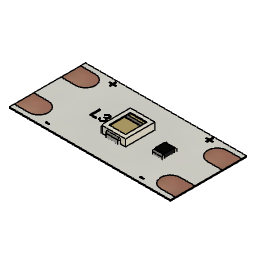
Shoulder LEDs v17 (Autodesk Fusion 360 archive; units mm, degrees)
design "LED D100"
Autodesk Fusion 360 part; units mm, degrees
sketch "Sketch1" plane through (0, 0, 0) normal (0, 0, 1) x (1, 0, 0)
  line L0 (0, 0) -> (16.5, 0)
  line L1 (16.5, 0) -> (16.5, 7.8)
  line L2 (0, 0) -> (0, 7.8)
  line L3 (16.5, 7.8) -> (0, 7.8)
  line L4 (8.25, 7.8) -> (8.25, 0) construction
  line L5 (0, 3.9) -> (16.5, 3.9) construction
  line L6 (8.25, 3.9) -> (8.25, 5.4) construction
  line L7 (8.25, 5.4) -> (8.25, 2.4) construction
  line L8 (8.25, 5.4) -> (7, 5.4) construction
  line L9 (7, 5.4) -> (9.5, 5.4)
  line L10 (9.5, 5.4) -> (9.5, 2.4)
  line L11 (9.5, 2.4) -> (7, 2.4)
  line L12 (7, 2.4) -> (7, 5.4)
  line L13 (7, 2.4) -> (9.5, 5.4) construction
  line L14 (7, 2.4) -> (7.064, 2.4768) construction
  line L15 (7.064, 2.4768) -> (7.1562, 2.4)
  line L16 (7.1562, 2.4) -> (7, 2.5302)
  line L17 (9.5, 3.9) -> (11.5, 3.9) construction
  line L18 (11.5, 3.9) -> (11.5, 4.65)
  line L19 (11.5, 4.65) -> (11.5, 3.15)
  line L20 (11.5, 3.15) -> (12.5, 3.15)
  line L21 (12.5, 3.15) -> (12.5, 4.65)
  line L22 (12.5, 4.65) -> (11.5, 4.65)
  line L23 (11.5, 3.15) -> (11.5, 3.4)
  line L24 (11.5, 4.65) -> (11.5, 4.4)
  line L25 (11.5, 4.4) -> (12.5, 4.4)
  line L26 (11.5, 3.4) -> (12.5, 3.4)
  line L27 (0, 7.8) -> (0, 7.3)
  line L28 (0, 7.3) -> (0, 5.3)
  line L29 (0, 0) -> (0, 0.5)
  line L30 (0, 0.5) -> (0, 2.5)
  line L31 (0, 7.3) -> (2.5, 7.3)
  line L32 (0, 0.5) -> (2.5, 0.5)
  line L33 (0, 2.5) -> (2.5, 2.5)
  line L34 (0, 5.3) -> (2.5, 5.3)
  line L35 (2.5, 0.5) -> (1.5, 0.5) construction
  line L36 (1.5, 0.5) -> (1.5, 7.3) construction
  line L37 (1.5, 5.3) -> (1.5, 7.3) construction
  circle A0 centre (1.5, 6.3) radius 1
  line L38 (1.5, 0.5) -> (1.5, 2.5) construction
  circle A1 centre (1.5, 1.5) radius 1
  line L39 (2.5, 0.5) -> (16.5, 0.5) construction
  line L40 (2.5, 5.3) -> (16.5, 5.3) construction
  line L41 (2.5, 7.3) -> (16.5, 7.3) construction
  line L42 (2.5, 2.5) -> (16.5, 2.5) construction
  line L43 (16.5, 0.5) -> (14, 0.5)
  line L44 (14, 0.5) -> (14, 7.8) construction
  line L45 (16.5, 7.3) -> (14, 7.3)
  line L46 (16.5, 5.3) -> (14, 5.3)
  line L47 (16.5, 2.5) -> (14, 2.5)
  line L48 (14, 2.5) -> (15, 2.5) construction
  line L49 (15, 2.5) -> (15, 0.5) construction
  line L50 (15, 2.5) -> (15, 7.3) construction
  line L51 (15, 7.3) -> (15, 5.3) construction
  circle A2 centre (15, 1.5) radius 1
  circle A3 centre (15, 6.3) radius 1
  line L52 (8.25, 2.4) -> (8.25, 2.25) construction
  line L53 (8.25, 2.25) -> (7.5, 2.25)
  line L54 (7.5, 2.25) -> (9, 2.25)
  line L55 (9, 2.25) -> (9, 5.4) construction
  line L56 (9, 5.4) -> (9, 5.55) construction
  line L57 (9, 5.55) -> (7.5, 5.55)
  line L58 (7.5, 2.25) -> (7.65, 2.25) construction
  line L59 (7.65, 2.25) -> (7.65, 2.4) construction
  circle A4 centre (7.65, 2.4) radius 0.15
  line L60 (9, 2.4) -> (8.85, 2.4) construction
  circle A5 centre (8.85, 2.4) radius 0.15
  line L61 (8.85, 2.4) -> (8.85, 5.4) construction
  line L62 (7.65, 2.4) -> (7.625, 5.4) construction
  circle A6 centre (7.625, 5.4) radius 0.15
  circle A7 centre (8.85, 5.4) radius 0.15
  dimension "d1" = 16.5
  dimension "d2" = 7.8
  dimension "d4" = 3
  dimension "d8" = 2.5
  dimension "d13" = 0.1
  dimension "d16" = 2
  dimension "d18" = 1.5
  dimension "d19" = 1
  dimension "d30" = 0.5
  dimension "d31" = 2
  dimension "d32" = 0.5
  dimension "d33" = 2
  dimension "d34" = 2.5
  dimension "d35" = 2.5
  dimension "d36" = 1
  dimension "d37" = 2
  dimension "d38" = 2.5
  dimension "d39" = 1
  dimension "d40" = 2
  dimension "d41" = 2
  dimension "d44" = 0.15
  dimension "d45" = 0.15
  dimension "d46" = 1.5
  dimension "d47" = 0.15
  dimension "d48" = 0.15
  dimension "d49" = 0.3
  dimension "d50" = 0.3
  dimension "d51" = 0.3
  constraint coincident L0.start L2.start
  constraint horizontal L0
  constraint perpendicular L0 L1
  constraint perpendicular L0 L2
  constraint perpendicular L2 L3
  constraint midpoint L3 L4.start
  constraint midpoint L0 L4.end
  constraint midpoint L2 L5.start
  constraint midpoint L1 L5.end
  constraint midpoint L5 L6.start
  constraint perpendicular L5 L6
  constraint perpendicular L5 L7
  constraint perpendicular L4 L8
  constraint parallel L8 L9
  constraint perpendicular L5 L10
  constraint perpendicular L10 L11
  constraint parallel L13 L14
  constraint coincident L11 L15.end
  constraint perpendicular L13 L15
  constraint coincident L12 L16.end
  constraint perpendicular L13 L16
  constraint midpoint L10 L17.start
  constraint perpendicular L10 L17
  constraint perpendicular L17 L18
  constraint perpendicular L5 L19
  constraint perpendicular L19 L20
  constraint perpendicular L20 L21
  constraint perpendicular L20 L23
  constraint perpendicular L22 L24
  constraint coincident L21 L25.end
  constraint perpendicular L21 L25
  constraint coincident L21 L26.end
  constraint perpendicular L21 L26
  constraint perpendicular L3 L27
  constraint parallel L2 L28
  constraint perpendicular L0 L29
  constraint parallel L2 L30
  constraint perpendicular L2 L31
  constraint perpendicular L30 L32
  constraint perpendicular L30 L33
  constraint perpendicular L2 L34
  constraint parallel L32 L35
  constraint coincident L31 L36.end
  constraint perpendicular L31 L36
  constraint coincident L36 L37.start
  constraint coincident L34 L37.start
  constraint midpoint L37 A0.centre
  constraint coincident L37.start A0
  constraint coincident L36 L38.end
  constraint midpoint L38 A1.centre
  constraint coincident L1 L39.end
  constraint perpendicular L1 L39
  constraint coincident L1 L40.end
  constraint perpendicular L1 L40
  constraint coincident L1 L41.end
  constraint perpendicular L1 L41
  constraint coincident L1 L42.end
  constraint perpendicular L1 L42
  constraint perpendicular L1 L43
  constraint coincident L3 L44.end
  constraint perpendicular L3 L44
  constraint coincident L44 L45.end
  constraint coincident L41 L45.end
  constraint coincident L44 L46.end
  constraint coincident L40 L46.end
  constraint coincident L44 L47.end
  constraint coincident L42 L47.end
  constraint perpendicular L44 L48
  constraint coincident L43 L49.end
  constraint coincident L45 L50.end
  constraint coincident L46 L51.end
  constraint coincident L50 L51.end
  constraint midpoint L49 A2.centre
  constraint midpoint L51 A3.centre
  constraint perpendicular L11 L52
  constraint perpendicular L52 L53
  constraint perpendicular L52 L54
  constraint coincident L9 L55.end
  constraint perpendicular L9 L55
  constraint perpendicular L9 L56
  constraint perpendicular L56 L57
  constraint parallel L54 L58
  constraint coincident L11 L59.end
  constraint perpendicular L11 L59
  constraint coincident L59.end A4.centre
  constraint coincident L58.end A4
  constraint coincident L55 L60.start
  constraint coincident L11 L60.start
  constraint perpendicular L55 L60
  constraint coincident L60.end A5.centre
  constraint perpendicular L40 L61
  constraint midpoint L8 L62.end
  constraint coincident L62.end A6.centre
  constraint coincident L61.end A7.centre
  measures "d1" distance of L0.start L0.end
  measures "d2" distance of L0.end L1.end
  measures "d4" distance of L6.end L7.end
  measures "d8" distance of L10.end L11.end
  measures "d13" distance of L11.end L14.end
  measures "d16" distance of L17.start L17.end
  measures "d18" distance of L18.end L19.end
  measures "d19" distance of L19.end L20.end
  measures "d30" distance of L2.end L27.end
  measures "d31" distance of L27.end L28.end
  measures "d32" distance of L0.start L29.end
  measures "d33" distance of L29.end L30.end
  measures "d34" distance of L27.end L31.end
  measures "d35" distance of L29.end L32.end
  measures "d36" distance of L32.end L35.end
  measures "d37" diameter of A1
  measures "d38" distance of L39.end L43.end
  measures "d39" distance of L47.end L48.end
  measures "d40" diameter of A2
  measures "d41" diameter of A3
  measures "d44" distance of L7.end L52.end
  measures "d45" distance of L55.end L56.end
  measures "d46" distance of L56.end L57.end
  measures "d47" distance of L53.end L58.end
  measures "d48" distance of L60.start L60.end
  measures "d49" diameter of A5
  measures "d50" diameter of A6
  measures "d51" diameter of A7
extrude "Extrude8" add sketch "Sketch1" along normal blind 0.6 contours L9 A7 | L9 L57 A6 A7 | L9 A6 | L11 A5 | L11 L53 L54 A4 A5 | L11 A4 picked at (8.7907, 5.4648) picked at (7.6552, 5.4726) picked at (8.8359, 2.352) picked at (7.6439, 2.325) makes body 1 at (8, 2.4, 0.4) makes body 2 at (7.9833, 5.4, 0.4)
extrude "Extrude5" add sketch "Sketch1" along normal blind 0.45 separate body contours L18 L19 L21 L22 L24 L25 | L19 L20 L21 L23 L26 makes body 3 at (11.8333, 3.4, 0.15) makes body 4 at (11.8333, 4.4, 0.15)
extrude "Extrude4" add sketch "Sketch1" along normal blind 0.5 separate body contours L18 L19 L21 L25 L26 makes body 5
extrude "Extrude3" add sketch "Sketch1" along normal blind 0.7 separate body contours L11 L12 L15 L16 makes body 6
extrude "Extrude2" add sketch "Sketch1" along normal blind 0.8 separate body contours L9 A7 | L9 L10 L11 L12 L15 L16 A4 A5 A6 A7 | L9 A6 | L11 A5 | L11 A4 picked at (8.8017, 5.3778) picked at (7.669, 5.3354) picked at (8.875, 2.4433) picked at (7.6077, 2.4878) makes body 7
extrude "Extrude1" add sketch "Sketch1" along normal blind 0.1 separate body contours L0 L1 L2 L3 L27 L29 L31 L32 L33 L34 A0 A1 L43 L45 L46 L47 A2 A3 | L9 A7 | L9 L57 A6 A7 | L9 A6 | L11 A5 | L11 L53 L54 A4 A5 | L11 A4 | L18 L19 L21 L25 L26 | L18 L19 L21 L22 L24 L25 | L19 L20 L21 L23 L26 picked at (8.7907, 5.4648) picked at (7.6552, 5.4726) picked at (8.8359, 2.352) picked at (7.6439, 2.325) makes body 8
sketch "Sketch2" plane through (0, 0, 0.8) normal (0, 0, 1) x (-1, 0, 0)
  line L0 (-7.1562, -2.4) -> (-9.5, -2.4)
  line L1 (-9.5, -2.4) -> (-9.5, -5.4)
  line L2 (-9.5, -5.4) -> (-7, -5.4)
  line L3 (-7, -5.4) -> (-7, -2.5302)
  line L4 (-7, -2.5302) -> (-7.1562, -2.4)
  line L5 (-9.1, -5) -> (-7.4, -5)
  line L6 (-7.4, -5) -> (-7.4, -2.8)
  line L7 (-7.4, -2.8) -> (-9.1, -2.8)
  line L8 (-9.1, -2.8) -> (-9.1, -5)
  line L9 (-9.1, -5) -> (-9.1, -4.7)
  line L10 (-9.1, -4.7) -> (-7.4, -4.7)
  line L11 (-7.4, -4.7) -> (-7.4, -4.4)
  line L12 (-7.4, -4.4) -> (-9.1, -4.4)
  dimension "d27" = -0.4
  dimension "d82" = 0.3
  dimension "d83" = 0.3
  constraint perpendicular L5 L9
  constraint coincident L6 L10.end
  constraint perpendicular L6 L10
  constraint perpendicular L10 L11
  constraint coincident L8 L12.end
  constraint perpendicular L8 L12
  measures "d82" distance of L5.start L9.end
  measures "d83" distance of L10.end L11.end
extrude "Extrude17" cut sketch "Sketch2" against normal blind 0.05 contours L6 L8 L10 L11 L12 bodies 7
extrude "Extrude16" cut sketch "Sketch2" against normal blind 0.1 contours L5 L6 L8 L9 L10 | L6 L7 L8 L12 bodies 7
extrude "Extrude7" add sketch "Sketch1" along normal blind 0.09 contours L2 L30 L32 L33 A1 | L1 L43 L47 A2 | A1 | A2 | L2 L28 L31 L34 A0 | L1 L45 L46 A3 | A0 | A3 bodies 8
fillet "Fillet1" radius 0.15 3 edges at (7.5439, 2.2939, 0.6) (8.25, 2.25, 0.6) (8.9561, 2.2939, 0.6) on bodies 1
fillet "Fillet2" radius 0.15 3 edges at (8.9561, 5.5061, 0.6) (8.2375, 5.55, 0.6) (7.5189, 5.5061, 0.6) on bodies 2
fillet "Fillet3" radius 0.15 2 edges at (12, 3.15, 0.45) (12, 4.65, 0.45) on bodies 3 4
sketch "Sketch3" plane through (0, 0, 0.1) normal (0, 0, 1) x (-1, 0, 0)
  line L0 (-9.5, -2.4) -> (-7, -2.4)
  line L1 (-7, -2.4) -> (-7, -5.4)
  line L2 (-7, -5.4) -> (-9.5, -5.4)
  line L3 (-9.5, -5.4) -> (-9.5, -2.4)
  line L4 (-16.5, -7.8) -> (0, -7.8)
  line L5 (0, -7.8) -> (0, -7.3)
  line L6 (0, -7.3) -> (-1.5, -7.3)
  arc A0 (-1.5, -5.3) -> (-1.5, -7.3) centre (-1.5, -6.3) ccw
  line L7 (-1.5, -5.3) -> (0, -5.3)
  line L8 (0, -5.3) -> (0, -2.5)
  line L9 (0, -2.5) -> (-1.4999, -2.5)
  arc A1 (-1.5, -0.5) -> (-1.4999, -2.5) centre (-1.5, -1.5) ccw
  line L10 (-1.5, -0.5) -> (0, -0.5)
  line L11 (0, -0.5) -> (0, 0)
  line L12 (0, 0) -> (-16.5, 0)
  line L13 (-16.5, 0) -> (-16.5, -0.5)
  line L14 (-16.5, -0.5) -> (-15.0001, -0.5)
  arc A2 (-15, -2.5) -> (-15.0001, -0.5) centre (-15, -1.5) ccw
  line L15 (-15, -2.5) -> (-16.5, -2.5)
  line L16 (-16.5, -2.5) -> (-16.5, -5.3)
  line L17 (-16.5, -5.3) -> (-15.0003, -5.3)
  arc A3 (-15, -7.3) -> (-15.0003, -5.3) centre (-15, -6.3) ccw
  line L18 (-15, -7.3) -> (-16.5, -7.3)
  line L19 (-16.5, -7.3) -> (-16.5, -7.8)
  line L20 (-2.9593, -6.3608) -> (-4.4543, -6.3608) construction
  line L21 (-4.4543, -6.3608) -> (-4.4543, -7.6424) construction
  line L22 (-4.4543, -7.6424) -> (-2.9593, -7.6424) construction
  line L23 (-2.9593, -7.6424) -> (-2.9593, -6.3608) construction
  dimension "d60" = 1
  text T0 "+\n" font "Arial" height 1 align left top in box 1.4949 x 1.2816 at (-2.9593, -6.3608) x (-1, 0) y (0, -1) spacing 1 kerned
extrude "Extrude9" add sketch "Sketch3" along normal blind 0.01 text T0 bodies 8
sketch "Sketch4" plane through (0, 0, 0.1) normal (0, 0, 1) x (-1, 0, 0)
  line L0 (-3.2315, -6.9814) -> (-3.2315, -7.2556)
  line L1 (-3.2315, -7.2556) -> (-2.9593, -7.2556)
  line L2 (-2.9593, -7.2556) -> (-2.9593, -7.3702)
  line L3 (-2.9593, -7.3702) -> (-3.2315, -7.3702)
  line L4 (-3.2315, -7.3702) -> (-3.2315, -7.6424)
  line L5 (-3.2315, -7.6424) -> (-3.3474, -7.6424)
  line L6 (-3.3474, -7.6424) -> (-3.3474, -7.3702)
  line L7 (-3.3474, -7.3702) -> (-3.6196, -7.3702)
  line L8 (-3.6196, -7.3702) -> (-3.6196, -7.2556)
  line L9 (-3.6196, -7.2556) -> (-3.3474, -7.2556)
  line L10 (-3.3474, -7.2556) -> (-3.3474, -6.9814)
  line L11 (-3.3474, -6.9814) -> (-3.2315, -6.9814)
  line L12 (-9.5, -2.4) -> (-7, -2.4)
  line L13 (-7, -2.4) -> (-7, -5.4)
  line L14 (-7, -5.4) -> (-9.5, -5.4)
  line L15 (-9.5, -5.4) -> (-9.5, -2.4)
  line L16 (-16.5, -7.8) -> (0, -7.8)
  line L17 (0, -7.8) -> (0, -7.3)
  line L18 (0, -7.3) -> (-1.5, -7.3)
  arc A0 (-1.5, -5.3) -> (-1.5, -7.3) centre (-1.5, -6.3) ccw
  line L19 (-1.5, -5.3) -> (0, -5.3)
  line L20 (0, -5.3) -> (0, -2.5)
  line L21 (0, -2.5) -> (-1.4999, -2.5)
  arc A1 (-1.5, -0.5) -> (-1.4999, -2.5) centre (-1.5, -1.5) ccw
  line L22 (-1.5, -0.5) -> (0, -0.5)
  line L23 (0, -0.5) -> (0, 0)
  line L24 (0, 0) -> (-16.5, 0)
  line L25 (-16.5, 0) -> (-16.5, -0.5)
  line L26 (-16.5, -0.5) -> (-15.0001, -0.5)
  arc A2 (-15, -2.5) -> (-15.0001, -0.5) centre (-15, -1.5) ccw
  line L27 (-15, -2.5) -> (-16.5, -2.5)
  line L28 (-16.5, -2.5) -> (-16.5, -5.3)
  line L29 (-16.5, -5.3) -> (-15.0003, -5.3)
  arc A3 (-15, -7.3) -> (-15.0003, -5.3) centre (-15, -6.3) ccw
  line L30 (-15, -7.3) -> (-16.5, -7.3)
  line L31 (-16.5, -7.3) -> (-16.5, -7.8)
  line L32 (-2.5, -6.3) -> (-2.5, 0) construction
  line L33 (-2.5, -7.8) -> (-2.5, -6.3) construction
  line L34 (-3.2315, -7.3702) -> (-3.3474, -7.2556) construction
  line L35 (-3.2315, -7.2556) -> (-3.3474, -7.3702) construction
  line L36 (-3.2895, -7.3129) -> (-2.5, -7.3129) construction
  line L37 (-3.2895, -7.3129) -> (-3.2895, 0) construction
  line L38 (-3.2895, -7.3129) -> (-3.2895, -7.8) construction
  line L39 (-3.2895, 0) -> (-3.2895, -0.5) construction
  line L40 (-3.2895, -0.5) -> (-3.5356, -0.5) construction
  line L41 (-3.5356, -0.5) -> (-3.5356, -0.741) construction
  line L42 (-3.5356, -0.741) -> (-3.2895, -0.741) construction
  line L43 (-3.2895, -0.741) -> (-3.2895, -0.5) construction
  line L44 (-14.0097, -7.8) -> (-14.0097, 0) construction
  line L45 (-14.0097, -7.8) -> (-13.2202, -7.8) construction
  line L46 (-13.2202, -7.8) -> (-13.2202, -7.3129) construction
  line L47 (-13.2202, -7.3129) -> (-13.2202, -7.5565)
  line L48 (-12.9907, -7.0628) -> (-13.3962, -7.0629) construction
  line L49 (-13.3962, -7.0629) -> (-13.3961, -7.5443) construction
  line L50 (-13.3961, -7.5443) -> (-12.9906, -7.5442) construction
  line L51 (-12.9906, -7.5442) -> (-12.9907, -7.0628) construction
  line L52 (-13.3961, -7.5443) -> (-13.3961, 0) construction
  line L53 (-13.3961, 0) -> (-13.3961, -0.4871) construction
  line L54 (-12.7786, -0.1002) -> (-13.3961, -0.1002) construction
  line L55 (-13.3961, -0.1002) -> (-13.3961, -0.5713) construction
  line L56 (-13.3961, -0.5713) -> (-12.7786, -0.5713) construction
  line L57 (-12.7786, -0.5713) -> (-12.7786, -0.1002) construction
  line L58 (-5.0528, -3.3) -> (-6.7528, -3.3) construction
  line L59 (-6.7528, -3.3) -> (-6.7528, -4.5) construction
  line L60 (-6.7528, -4.5) -> (-5.0528, -4.5) construction
  line L61 (-5.0528, -4.5) -> (-5.0528, -3.3) construction
  dimension "d63" = 0.5
  dimension "d67" = 1
  dimension "d70" = 0.7895
  dimension "d71" = 0.4871
  dimension "d72" = 0.7895
  dimension "d73" = 0.4871
  dimension "d74" = 1
  dimension "d75" = 0.4871
  dimension "d76" = 1
  dimension "d79" = 1
  text T0 "-" font "Arial" height 1 align centre middle in box 0.2462 x 0.241 at (-3.2895, -0.5) x (-1, 0) y (0, -1) spacing 1 kerned
  text T1 "+" font "Arial" height 1 align centre middle in box 0.4055 x 0.4815 at (-12.9907, -7.0628) x (-1, -0.000239) y (0.000239, -1) spacing 1 kerned
  text T2 "-" font "Arial" height 1 align centre middle in box 0.6174 x 0.4711 at (-12.7786, -0.1002) x (-1, 0) y (0, -1) spacing 1 kerned
  text T3 "L30" font "Arial" height 1 align centre middle in box 1.7 x 1.2 at (-5.0528, -3.3) x (-1, 0) y (0, -1) spacing 1 kerned
  constraint midpoint A0 L32.start
  constraint coincident L24 L32.end
  constraint tangent A0 L32
  constraint perpendicular L24 L32
  constraint coincident L16 L33.start
  constraint tangent A0 L33
  constraint coincident L3.end L4.start
  constraint coincident L9.end L10.start
  constraint coincident L0.end L1.start
  constraint coincident L6.end L7.start
  constraint midpoint L35 L36.start
  constraint coincident L33 L36.end
  constraint perpendicular L33 L36
  constraint coincident L24 L37.end
  constraint perpendicular L24 L37
  constraint coincident L16 L38.end
  constraint perpendicular L16 L38
  constraint perpendicular L24 L39
  constraint coincident L39.end
  constraint coincident L16 L44.start
  constraint coincident L24 L44.end
  constraint perpendicular L24 L44
  constraint coincident L16 L45.end
  constraint perpendicular L44 L45
  constraint perpendicular L45 L46
  constraint midpoint L46 L47.end
  constraint coincident L49.end
  constraint coincident L24 L52.end
  constraint perpendicular L24 L52
  constraint coincident L52 L53.end
  constraint coincident L53
  measures "d63" distance of L37.end L39.end
  measures "d70" distance of L36.start L36.end
  measures "d71" distance of L36.start L38.end
  measures "d72" distance of L44.start L45.end
  measures "d73" distance of L45.end L46.end
  measures "d75" distance of L52.end L53.end
extrude "Extrude13" add sketch "Sketch4" along normal blind 0.01 text T3 bodies 8
extrude "Extrude12" add sketch "Sketch4" along normal blind 0.01 text T2 T1 bodies 8
extrude "Extrude11" add sketch "Sketch4" along normal blind 0.01 text T0 bodies 8
equation "d72 = d70"
equation "d75 = d73"
